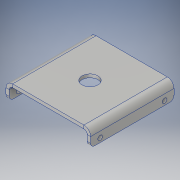
# Autodesk Inventor part: Support Plate
Saved by Autodesk Inventor 2019.4 (Build 234330000, 330)
## iProperties
Created: 2019-11-30
Part Number: Support Plate
Material: Aluminum 6061
Document SubType Name: Sheet Metal
Designer: admin
Density: 2.7 g/cm^3
Sheet Metal Rule: Default_mm
Appearance: Aluminum - Flat
Mass: 138.618 g
Surface Area: 274.967 cm^2
Volume: 51.3398 cm^3
Author: admin
Autodesk Inventor part; units mm, degrees
ref_plane "YZ Plane" through (0, 0, 0) normal (1, 0, 0) x (0, 1, 0)
ref_plane "XZ Plane" through (0, 0, 0) normal (0, 1, 0) x (-1, 0, 0)
ref_plane "XY Plane" through (0, 0, 0) normal (0, 0, 1) x (1, 0, 0)
sketch "Sketch1" plane through (0, 0, 0) normal (0, 0, 1) x (1, 0, 0)
  line L0 (0, 0) -> (0, 20)
  line L1 (0, 20) -> (101.5, 20)
  line L2 (101.5, 20) -> (101.5, 0)
  dimension "d0" = 101.5
  dimension "d1" = 20
  dimension "d2" = 20
  measures "d0" distance of L0.end L1.end
  measures "d1" distance of L0.start L0.end
  measures "d2" distance of L1.end L2.end
contour flange "Contour Flange1" sketch "Sketch1" thickness 4 bend radius 4 width 100 along (0, 0, 1) mid plane no both sides no wall seen from (0, 10, 0) lies toward (1, 0, 0) curves L0 L1 L2
bend "Bend1"
corner "Corner1"
sketch "Sketch2" plane through (101.5, 0, 100) normal (1, 0, 0) x (0, 0, -1)
  circle A0 centre (11.3565, 5) radius 2.75
  circle A1 centre (88.6435, 5) radius 2.75
  line L0 (88.6435, 5) -> (11.3565, 5) construction
  line L1 (50, 5) -> (50, 0) construction
  line L2 (100, 0) -> (0, 0) projected
  dimension "d14" = 5.5
  dimension "d15" = 5.5
  dimension "d16" = 5
  constraints: 4 end point, 2 centre point, 2 midpoint, 1 horizontal, 1 vertical
  measures "d14" diameter of A0
  measures "d15" diameter of A1
  measures "d16" distance from line of L2 L0.start
extrude "Extrusion1" cut sketch "Sketch2" against normal through all
fillet "Fillet1" radius 5 4 edges at (99.5, 0, 100) (99.5, 0, 0) (2, 0, 100) (2, 0, 0)
sketch "Sketch3" plane through (8, 20, 0) normal (0, 1, 0) x (1, 0, 0)
  line L0 (0, -100) -> (85.5, -100)
  line L1 (85.5, -100) -> (85.5, 0)
  line L2 (85.5, 0) -> (0, 0)
  line L3 (0, 0) -> (0, -100)
  line L4 (0, -100) -> (85.5, 0) construction
  line L5 (85.5, -100) -> (0, 0) construction
  line L6 (0, 0) -> (85.5, 0) projected
  line L7 (85.5, 0) -> (85.5, -100) projected
  line L8 (85.5, -100) -> (0, -100) projected
  line L9 (0, 0) -> (0, -100) projected
  circle A0 centre (42.75, -50) radius 9.5
  point P0 (-8, 0)
  point P1 (42.75, -50)
  dimension "d20" = 19
  constraints: 12 end point, 4 collinear, 2 midpoint, 2 parallel, 1 centre point, 1 coincident, 1 horizontal, 1 perpendicular
  measures "d20" diameter of A0
extrude "Extrusion2" cut sketch "Sketch3" against normal blind 10 contours A0
equation "\"d2\" = d1"
equation "\"d3\" = Thickness"
equation "\"d4\" = BendReliefWidth"
equation "\"d5\" = BendReliefDepth"
equation "\"d6\" = MinimumRemnant"
equation "\"d7\" = TransitionRadius"
equation "\"d9\" = BendRadius"
equation "\"d11\" = CornerReliefSize"
equation "\"d12\" = GapSize"
equation "\"d13\" = JacobiRadiusSize"
equation "\"BendRadius\" = Thickness"
equation "\"BendReliefWidth\" = Thickness"
equation "\"BendReliefDepth\" = 0.5 * Thickness"
equation "\"CornerReliefSize\" = 4 * Thickness"
equation "\"MinimumRemnant\" = 2 * Thickness"
equation "\"TransitionRadius\" = BendRadius"
equation "\"JacobiRadiusSize\" = BendRadius"
equation "\"GapSize\" = Thickness"
equation "\"Thickness\" = 4"
body "Solid1"
